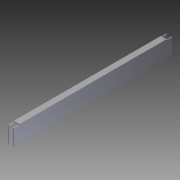
# Autodesk Inventor part: frame box 1 by 3
Saved by Autodesk Inventor 2012 (Build 160160000, 160)
## iProperties
Created: 2013-09-01
Part Number: frame box 1 by 3
Material: Default
Document SubType Name: Modeling
Designer: Bryce
Density: 1 g/cm^3
Author: Bryce
Autodesk Inventor part; units mm, degrees
ref_plane "YZ Plane" through (0, 0, 0) normal (1, 0, 0) x (0, 1, 0)
ref_plane "XZ Plane" through (0, 0, 0) normal (0, 1, 0) x (-1, 0, 0)
ref_plane "XY Plane" through (0, 0, 0) normal (0, 0, 1) x (1, 0, 0)
sketch "Sketch1" plane through (0, 0, 0) normal (0, 0, 1) x (1, 0, 0)
  line L0 (0, 0) -> (25.4, 0)
  line L1 (25.4, 0) -> (25.4, 76.2)
  line L2 (25.4, 76.2) -> (0, 76.2)
  line L3 (0, 76.2) -> (0, 0)
  line L4 (3.175, 3.175) -> (22.225, 3.175)
  line L5 (22.225, 3.175) -> (22.225, 73.025)
  line L6 (22.225, 73.025) -> (3.175, 73.025)
  line L7 (3.175, 73.025) -> (3.175, 3.175)
  dimension "d0" = 25.4
  dimension "d1" = 76.2
  dimension "d2" = 3.175
  dimension "d3" = 3.175
  dimension "d4" = 3.175
  dimension "d5" = 3.175
  constraints: 16 end point, 4 parallel, 2 horizontal, 2 perpendicular
  measures "d0" distance of L1.end L2.end
  measures "d1" distance of L2.end L0.start
  measures "d2" distance between parallel lines of L0 L4
  measures "d3" distance between parallel lines of L7 L3
  measures "d4" distance between parallel lines of L6 L2
  measures "d5" distance between parallel lines of L1 L5
extrude "Extrusion1" add sketch "Sketch1" along normal blind 704.85
sketch "Sketch2" plane through (0, 76.2, 0) normal (0, 1, 0) x (1, 0, 0)
  line L0 (0, -704.85) -> (25.4, -704.85) projected
  line L1 (25.4, 0) -> (25.4, -704.85) projected
  line L2 (25.4, 0) -> (0, 0) projected
  line L3 (0, 0) -> (0, -704.85) projected
  line L4 (0, -25.4) -> (25.4, -25.4)
  line L5 (0, -679.45) -> (25.4, -679.45)
  dimension "d8" = 25.4
  dimension "d9" = 25.4
  constraints: 4 end point, 4 point on line, 2 perpendicular
  measures "d8" distance between parallel lines of L0 L5
  measures "d9" distance between parallel lines of L4 L2
extrude "Extrusion2" cut sketch "Sketch2" against normal blind 3.175 contours L3 L5 L1 L0 | L3 L2 L1 L4
sketch "Sketch3" plane through (0, 0, 0) normal (0, -1, 0) x (1, 0, 0)
  line L0 (25.4, 704.85) -> (0, 704.85) projected
  line L1 (0, 0) -> (0, 704.85) projected
  line L2 (0, 0) -> (25.4, 0) projected
  line L3 (25.4, 0) -> (25.4, 704.85) projected
  line L4 (0, 679.45) -> (25.4, 679.45)
  line L5 (0, 25.4) -> (25.4, 25.4)
  dimension "d12" = 25.4
  dimension "d13" = 25.4
  constraints: 4 end point, 4 point on line, 2 perpendicular
  measures "d12" distance between parallel lines of L2 L5
  measures "d13" distance between parallel lines of L4 L0
extrude "Extrusion3" cut sketch "Sketch3" against normal blind 3.175 contours L3 L4 L1 L0 | L3 L2 L1 L5
equation "\"d3\" = d2"
equation "\"d4\" = d3"
equation "\"d5\" = d4"
equation "\"d9\" = d8"
body "Solid1"
